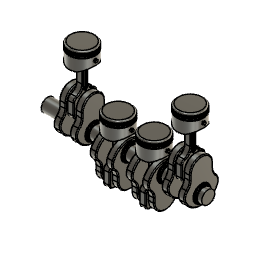
engine V4 (Autodesk Fusion 360 design; units mm, degrees)
Autodesk Fusion 360 part; units mm, degrees
note: some values were not read from the file. Set by a fixed rule: which face or edge a step refers to.
sketch "Sketch1" plane through (0, 0, 0) normal (0, 1, 0) x (1, 0, 0) in component "pistons"
  line L0 (0, 0) -> (40, 0)
  line L1 (40, 0) -> (40, -55)
  line L2 (40, -55) -> (0, -55)
  line L3 (0, -55) -> (0, 0)
  line L4 (40, -48) -> (36, -48)
  line L5 (36, -48) -> (36, -46)
  line L6 (36, -46) -> (40, -46)
  line L7 (40, -46) -> (40, -48)
  line L8 (40, -44) -> (36, -44)
  line L9 (36, -44) -> (36, -42)
  line L10 (36, -42) -> (40, -42)
  line L11 (40, -42) -> (40, -44)
  line L12 (40, -38) -> (36, -38)
  line L13 (36, -38) -> (36, -36)
  line L14 (36, -36) -> (40, -36)
  line L15 (40, -36) -> (40, -38)
  dimension "d1" = 40
  dimension "d2" = 55
  dimension "d3" = 2
  dimension "d4" = 2
  dimension "d5" = 2
  dimension "d6" = 7
  dimension "d7" = 4
  dimension "d8" = 4
  dimension "d9" = 4
  dimension "d10" = 2
  dimension "d11" = 4
  constraint horizontal L0
  constraint vertical L1
  constraint horizontal L2
  constraint vertical L3
  constraint coincident L0.start L3.end
  constraint horizontal L4
  constraint vertical L5
  constraint horizontal L6
  constraint vertical L7
  constraint coincident L1 L4.start
  constraint horizontal L8
  constraint vertical L9
  constraint horizontal L10
  constraint vertical L11
  constraint coincident L1 L8.start
  constraint horizontal L12
  constraint vertical L13
  constraint horizontal L14
  constraint vertical L15
  constraint coincident L1 L12.start
  measures "d1" distance of L0.start L0.end
  measures "d2" distance of L0.start L2.end
  measures "d3" distance of L4.end L5.end
  measures "d4" distance of L8.end L9.end
  measures "d5" distance of L12.end L13.end
  measures "d6" distance of L2 L4
  measures "d7" distance of L4.start L4.end
  measures "d8" distance of L8.start L8.end
  measures "d9" distance of L12.start L12.end
  measures "d10" distance of L6 L8
  measures "d11" distance of L10 L12
revolve "Revolve1" add sketch "Sketch1" angle 360 about axis through (0, 0, 55) along (0, 0, -1) contours L0 L1 L2 L3 L4 L5 L6 L8 L9 L10 L12 L13 L14 makes body 1 in component "pistons"
fillet "Fillet1" radius 5 1 edges at (-37.2931, -14.4646, 55) on bodies 1 in component "pistons"
sketch "Sketch2" plane through (0, 0, 0) normal (0, 0, -1) x (1, 0, 0) in component "pistons"
  circle A0 centre (0, 0) radius 40
  circle A1 centre (0, 0) radius 35
  dimension "d15" = 70
  constraint coincident A0.centre A1.centre
  measures "d15" diameter of A1
extrude "Extrude1" cut sketch "Sketch2" against normal blind 50 contours A1 bodies 1 in component "pistons"
sketch "Sketch3" plane through (0, 0, 0) normal (1, 0, 0) x (0, 1, 0) in component "pistons"
  line L0 (40, 0) -> (-40, 0)
  line L1 (40, 36) -> (-40, 36)
  line L2 (0, 0) -> (0, 10)
  arc A0 (35.5, 0) -> (-35.5, 0) centre (0, -58.0125) ccw
  circle A1 centre (0, 24) radius 5
  dimension "d18" = 10
  dimension "d19" = 10
  dimension "d20" = 4.5
  dimension "d21" = 4.5
  dimension "d22" = 24
  constraint coincident L2.start origin
  constraint perpendicular L0 L2
  constraint coincident L2.end A0
  constraint coincident L0 A0.start
  constraint coincident L0 A0.end
  measures "d18" distance of L2.start L2.end
  measures "d19" diameter of A1
  measures "d20" distance of L0.end A0.end
  measures "d21" distance of L0.start A0.start
  measures "d22" distance of L2.start A1.centre
extrude "Extrude2" cut sketch "Sketch3" along normal mid plane 160 bodies 1 in component "pistons"
pattern_linear "00000000-0000-0000-0000-000000000000" [suppressed] in component "piston"
sketch "Sketch1 (2)" plane through (0, 0, 0) normal (1, 0, 0) x (0, 1, 0) in component "Connecting Rod"
  circle A0 centre (0, 30) radius 5
  circle A1 centre (0, 30) radius 8.5
  circle A2 centre (0, -95) radius 22.5
  line L0 (8.5, 30) -> (8.5, -45)
  line L1 (0, -95) -> (36, -95)
  line L2 (36, -95) -> (36, -70)
  line L3 (36, -70) -> (33.5, -70)
  arc A3 (8.5, -45) -> (33.5, -70) centre (33.5, -45) ccw
  line L4 (0, -95) -> (0, -45) construction
  arc A4 (-33.5, -70) -> (-8.5, -45) centre (-33.5, -45) ccw
  line L5 (-36, -70) -> (-33.5, -70)
  line L6 (-36, -95) -> (-36, -70)
  line L7 (0, -95) -> (-36, -95)
  line L8 (-8.5, 30) -> (-8.5, -45)
  line L9 (-36, -95) -> (36, -95)
  line L10 (36, -95) -> (36, -127.5)
  line L11 (36, -127.5) -> (-36, -127.5)
  line L12 (-36, -127.5) -> (-36, -95)
  circle A5 centre (0, 15) radius 4.75
  circle A6 centre (0, -57.5) radius 4.75
  line L13 (-4.75, 15) -> (-4.75, -57.5)
  line L14 (4.75, 14.9999) -> (4.75, -57.5)
  dimension "d29" = 10
  dimension "d30" = 17
  dimension "d31" = 45
  dimension "d32" = 125
  dimension "d33" = 36
  dimension "d34" = 25
  dimension "d35" = 25
  dimension "d36" = 72
  dimension "d37" = 32.5
  dimension "d38" = 9.5
  dimension "d39" = 9.5
  dimension "d40" = 15
  dimension "d41" = 37.5
  constraint concentric A0 A1
  constraint coincident A1 L0.start
  constraint tangent A1 L0
  constraint vertical L0
  constraint coincident A2.centre L1.start
  constraint horizontal L1
  constraint perpendicular L1 L2
  constraint perpendicular L2 L3
  constraint tangent L0 A3
  constraint tangent L3 A3
  constraint perpendicular L1 L4
  constraint symmetric L0.start L4 L8.start
  constraint symmetric A2.centre L4 L1.start
  constraint symmetric L1.end L4 L6.start
  constraint symmetric L2.end L4 L5.start
  constraint symmetric L0.end L4 A4.end
  constraint symmetric L3.end L4 A4.start
  constraint symmetric A3 L4 A4
  constraint horizontal L9
  constraint vertical L10
  constraint horizontal L11
  constraint vertical L12
  constraint coincident A5 L13.start
  constraint coincident A6 L13.end
  constraint tangent A6 L13
  constraint parallel L8 L13
  constraint coincident A5 L14.start
  constraint coincident A6 L14.end
  constraint tangent A6 L14
  constraint parallel L0 L14
  measures "d29" diameter of A0
  measures "d30" diameter of A1
  measures "d31" diameter of A2
  measures "d32" distance of A0.centre A2.centre
  measures "d33" distance of A2.centre L1.end
  measures "d34" distance of L1.end L2.end
  measures "d35" radius of A3
  measures "d36" distance of L6.start L1.end
  measures "d37" distance of L6.start L11.end
  measures "d38" diameter of A5
  measures "d39" diameter of A6
  measures "d40" distance of A0.centre A5.centre
  measures "d41" distance of A2.centre A6.centre
extrude "Extrude1'" add sketch "Sketch1 (2)" along normal mid plane 20 separate body contours A1 | A1 A2 L0 L1 L2 L3 A3 A4 L5 L6 L7 L8 L9 | A2 L1 L7 L9 L10 L11 L12 makes body 2 in component "Connecting Rod"
extrude "Extrude2'" add sketch "Sketch1 (2)" along normal mid plane 10 contours A5 | A5 A6 L13 L14 | A6 bodies 2 in component "Connecting Rod"
fillet "Fillet1'" radius 12.5 4 edges at (0, 36, -70) (0, -36, -70) (0, 36, -127.5) (0, -36, -127.5) on bodies 2 in component "Connecting Rod"
fillet "Fillet2" radius 2.5 24 edges at (10, -8.5, -7.5) (10, -13.6044, -60.1383) (10, -33.4478, -73.573) (10, -36, -98.071) (10, -32.3388, -123.8388) (10, 0, -127.5) (10, 32.3388, -123.8388) (10, 36, -98.071) (10, 33.4478, -73.573) (10, 13.6044, -60.1383) (10, 8.5, -7.5) (10, 0, 38.5) (-10, 33.4478, -73.573) (-10, 36, -98.071) (-10, 32.3388, -123.8388) (-10, 0, -127.5) (-10, -32.3388, -123.8388) (-10, -36, -98.071) (-10, -33.4478, -73.573) (-10, -13.6044, -60.1383) (-10, -8.5, -7.5) (-10, 0, 38.5) (-10, 8.5, -7.5) (-10, 13.6044, -60.1383) on bodies 2 in component "Connecting Rod"
fillet "Fillet3" radius 1.5 16 edges at (5, 4.75, -21.2501) (5, 0, -62.25) (5, -4.75, -21.25) (5, 0.0001, 19.75) (10, 4.75, -21.2501) (10, 0, -62.25) (10, -4.75, -21.25) (10, 0.0001, 19.75) (-10, 4.75, -21.2501) (-10, 0.0001, 19.75) (-10, -4.75, -21.25) (-10, 0, -62.25) (-5, 4.75, -21.2501) (-5, 0.0001, 19.75) (-5, -4.75, -21.25) (-5, 0, -62.25) on bodies 2 in component "Connecting Rod"
cylinder "CylinderPrimitive1" add diameter 10 height 90 placed x (0, 0, -1) y (0, 1, 0) z (1, 0, 0) at (0, 0, 100) separate body makes body 3 in component "Pins (1)"
fillet "Fillet1''" radius 1.5 2 edges at (0, 1.8081, 104.6616) (90, -1.8081, 104.6616) on bodies 3 in component "Pins (1)"
pattern_linear "00000000-0000-0000-0000-000000000000'" [suppressed] in component "Pins"
sketch "Sketch1 (3)" plane through (0, 0, 0) normal (1, 0, 0) x (0, 1, 0) in component "Crank Shaft"
  circle A0 centre (0, -95) radius 22.5
  circle A1 centre (0, -95) radius 35
  circle A2 centre (0, -30.5) radius 20
  circle A3 centre (0, -30.5) radius 25
  arc A4 (55, -52.5) -> (-55, -52.5) centre (0, -52.5) ccw
  line L0 (35, -95) -> (35, -52.5)
  line L1 (-35, -95) -> (-35, -52.5)
  line L2 (-35, -52.5) -> (-55, -52.5)
  line L3 (35, -52.5) -> (55, -52.5)
  dimension "d69" = 70
  dimension "d74" = 42.5
  dimension "d75" = 40
  dimension "d76" = 50
  dimension "d77" = 22
  constraint concentric A0 A1
  constraint concentric A2 A3
  constraint coincident A1 L0.start
  constraint tangent A1 L0
  constraint coincident A1 L1.start
  constraint tangent A1 L1
  measures "d69" diameter of A1
  measures "d74" distance of A0.centre A4.centre
  measures "d75" diameter of A2
  measures "d76" diameter of A3
  measures "d77" distance of A2.centre A4.centre
extrude "Extrude1''" add sketch "Sketch1 (3)" along normal blind 20 from surface at 15 separate body contours A0 | A1 | A1 A4 L0 L1 L2 L3 | A2 | A3 makes body 4 in component "Crank Shaft"
extrude "Extrude2''" add sketch "Sketch1 (3)" along normal blind 20 from surface at 35 contours A2 bodies 4 in component "Crank Shaft"
extrude "Extrude3" add sketch "Sketch1 (3)" along normal blind 5 from surface at 35 contours A3 bodies 4 in component "Crank Shaft"
fillet "Fillet1'''" radius 30 2 edges at (25, -35, -52.5) (25, 35, -52.5) on bodies 4 in component "Crank Shaft"
fillet "Fillet2'" radius 25 2 edges at (25, 55, -52.5) (25, -55, -52.5) on bodies 4 in component "Crank Shaft"
fillet "Fillet3'" radius 2.5 16 edges at (35, -51.987, -45.6375) (35, -37.4915, -68.8142) (35, -35, -87.8921) (35, 0, -130) (35, 35, -87.8921) (35, 37.4915, -68.8142) (35, 51.987, -45.6375) (35, 0, 2.5) (15, -37.4915, -68.8142) (15, -35, -87.8921) (15, 0, -130) (15, 35, -87.8921) (15, 37.4915, -68.8142) (15, 51.987, -45.6375) (15, 0, 2.5) (15, -51.987, -45.6375) on bodies 4 in component "Crank Shaft"
fillet "Fillet4" radius 1.5 3 edges at (35, -23.3082, -21.4596) (40, -23.3082, -39.5404) (40, -18.6465, -37.7323) on bodies 4 in component "Crank Shaft"
mirror "Mirror1" about plane through (0, 0, 0) normal (1, 0, 0) of bodies 4 makes body 5 in component "Crank Shaft"
extrude "Extrude4" add sketch "Sketch1 (3)" along normal mid plane 30 contours A0 bodies 4 5 in component "Crank Shaft"
pattern_linear "R-Pattern1" count 4 spacing 110 along (-1, 0, 0) of bodies 4 makes body 6 at (-95, -26.5501, -48.8431) makes body 7 at (-205, -26.5501, -48.8431) makes body 8 at (-315, -26.5501, -48.8431) in component "Crank Shaft"
move_body "Move1" bodies 6 7 to x (1, 0, 0) y (0, -1, 0) z (0, 0, -1) at (0, 0, -61) in component "Crank Shaft"
combine "Combine1" operation add target body 7 tool bodies 8 6 4 in component "Crank Shaft"
extrude "Extrude5" add 1 faces at (-385, -0.7146, -25.2878) along direction (-1, 0, 0) blind 50 on bodies 7 bodies 7 in component "Crank Shaft"
sketch "Sketch1 (4)" plane through (-435, 0, 0) normal (-1, 0, 0) x (0, -1, 0)
  circle A0 centre (0, -30.5) radius 20
  circle A1 centre (0, -30.5) radius 37.5
  dimension "d105" = 75
  constraint concentric A0 A1
  measures "d105" diameter of A1
extrude "Extrude1'''" add sketch "Sketch1 (4)" against normal blind 20 separate body makes body 9 in component "Component"
pattern_linear "00000000-0000-0000-0000-000000000000''" [suppressed] in component "Connecting Rods"
sketch "Sketch2 (2)" plane through (0, 0, 190) normal (0, 0, 1) x (-1, 0, 0)
  circle A0 centre (219.9976, 0) radius 35
  line L0 (-113.2375, -187.2934) -> (555.2088, -187.2934)
  line L1 (555.2088, -187.2934) -> (555.2088, 234.2028)
  line L2 (555.2088, 234.2028) -> (-113.2375, 234.2028)
  line L3 (-113.2375, 234.2028) -> (-113.2375, -187.2934)
  circle A1 centre (329.9976, 0) radius 40
  circle A2 centre (219.9976, 0) radius 40
  circle A3 centre (110.0024, 0) radius 40
  circle A4 centre (-0.0024, 0) radius 40
  constraint horizontal L0
  constraint vertical L1
  constraint horizontal L2
  constraint vertical L3
extrude "Extrude1''''" add sketch "Sketch2 (2)" along normal blind 25 separate body contours L0 L1 L2 L3 makes body 10 in component "Component'"
component "piston" placed x (1, 0, 0) y (0, 1, 0) z (0, 0, 1) at (0, 0, 0)
component "Connecting Rods" placed x (1, 0, 0) y (0, 1, 0) z (0, 0, 1) at (0, 0, 0)
component "Pins" placed x (1, 0, 0) y (0, 1, 0) z (0, 0, 1) at (0, 0, 0)
component "Crank Shaft" placed x (1, 0, 0) y (0, -1, 0) z (0, 0, -1) at (0, 0, -61)
component "Component" placed x (1, 0, 0) y (0, 1, 0) z (0, 0, 1) at (0, 0, 0)
component "Component'" placed x (1, 0, 0) y (0, 1, 0) z (0, 0, 1) at (0, 0, 0)
component "pistons" placed x (1, 0, 0) y (0, 1, 0) z (0, 0, 1) at (-329.9976, 0, 135) in component "piston"
component "pistons" placed x (1, 0, 0) y (0, 1, 0) z (0, 0, 1) at (-219.9976, 0, 6) in component "piston"
component "pistons" placed x (1, 0, 0) y (0, 1, 0) z (0, 0, 1) at (-110.0024, 0, 6) in component "piston"
component "pistons" placed x (1, 0, 0) y (0, 1, 0) z (0, 0, 1) at (0.0024, 0, 135) in component "piston"
component "Connecting Rod" placed x (1, 0, 0) y (0, 1, 0) z (0, 0, 1) at (0, 0, 129) in component "Connecting Rods"
component "Connecting Rod" placed x (1, 0, 0) y (0, 1, 0) z (0, 0, 1) at (-110, 0, 0) in component "Connecting Rods"
component "Connecting Rod" placed x (1, 0, 0) y (0, 1, 0) z (0, 0, 1) at (-220, 0, 0) in component "Connecting Rods"
component "Connecting Rod" placed x (1, 0, 0) y (0, 1, 0) z (0, 0, 1) at (-330, 0, 129) in component "Connecting Rods"
component "Pins (1)" placed x (1, 0, 0) y (0, 1, 0) z (0, 0, 1) at (-45, 0, 59) in component "Pins"
component "Pins (1)" placed x (1, 0, 0) y (0, 1, 0) z (0, 0, 1) at (-155, 0, -70) in component "Pins"
component "Pins (1)" placed x (1, 0, 0) y (0, 1, 0) z (0, 0, 1) at (-265, 0, -70) in component "Pins"
component "Pins (1)" placed x (1, 0, 0) y (0, 1, 0) z (0, 0, 1) at (-375, 0, 59) in component "Pins"
